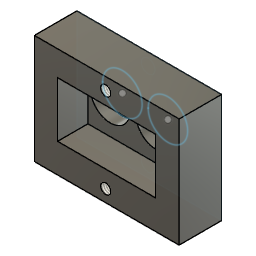
LP8-TAPA v5 (Autodesk Fusion 360 design; units mm, degrees)
Autodesk Fusion 360 part; units mm, degrees
sketch "Boceto1" plane through (0, 0, 0) normal (0, 0, 1) x (1, 0, 0)
  line L0 (0, 0) -> (47.682, 0)
  line L1 (47.682, 0) -> (47.682, 36)
  line L2 (47.682, 36) -> (0, 36)
  line L3 (0, 36) -> (0, 0)
  line L4 (4.2944, 26.5117) -> (42.5805, 26.5117)
  line L5 (42.5805, 26.5117) -> (42.5805, 9.2899)
  line L6 (42.5805, 9.2899) -> (4.2944, 9.2899)
  line L7 (4.2944, 9.2899) -> (4.2944, 26.5117)
  circle A0 centre (23.5, 32) radius 2.25
  circle A1 centre (23.5, 4) radius 2.25
  dimension "d8" = 4.5
  dimension "d10" = 4.5
  constraint horizontal L0
  constraint vertical L1
  constraint horizontal L2
  constraint vertical L3
  constraint coincident L0.start L3.end
  constraint horizontal L4
  constraint vertical L5
  constraint horizontal L6
  constraint vertical L7
  measures "d8" diameter of A0
  measures "d10" diameter of A1
extrude "Extruir1" add sketch "Boceto1" against normal blind 14 contours L0 L1 L2 L3 | L4 L5 L6 L7
sketch "Boceto2" plane through (0, 0, 0) normal (0, 0, 1) x (1, 0, 0)
  circle A0 centre (23.5, 4) radius 2.25
  circle A1 centre (23.5, 32) radius 2.25
  line L0 (0, 36) -> (0, 0)
  line L1 (0, 0) -> (47.682, 0)
  line L2 (47.682, 0) -> (47.682, 36)
  line L3 (47.682, 36) -> (0, 36)
  line L4 (7.6346, 27.7605) -> (39.9467, 27.7605)
  line L5 (39.9467, 27.7605) -> (39.9467, 9.5968)
  line L6 (39.9467, 9.5968) -> (7.6346, 9.5968)
  line L7 (7.6346, 9.5968) -> (7.6346, 27.7605)
  constraint horizontal L4
  constraint vertical L5
  constraint horizontal L6
  constraint vertical L7
extrude "Extruir2" cut sketch "Boceto2" against normal blind 10 contours L4 L5 L6 L7
sketch "Boceto3" plane through (0, 0, -14) normal (0, 0, -1) x (-1, 0, 0)
  circle A0 centre (-23.5, 4) radius 2.25
  circle A1 centre (-23.5, 32) radius 2.25
  line L0 (0, 0) -> (0, 36)
  line L1 (0, 36) -> (-47.682, 36)
  line L2 (-47.682, 36) -> (-47.682, 0)
  line L3 (-47.682, 0) -> (0, 0)
  circle A2 centre (-30, 20) radius 6.5
  circle A3 centre (-15, 20) radius 6.5
  dimension "d25" = 13
  dimension "d26" = 13
  measures "d25" diameter of A2
  measures "d26" diameter of A3
extrude "Extruir3" cut sketch "Boceto3" against normal blind 25 contours A2 | A3
thread "Rosca1" "ISO Metric profile 4.0 M4x0.7 M4x0.7 6H" major diameter 4.1095 minor diameter 3.332 pitch 0.7 angle 60 resizes the face on face at (25.7388, 31.776, -9.3333)
thread "Rosca2" "ISO Metric profile 4.0 M4x0.7 M4x0.7 6H" major diameter 4.1095 minor diameter 3.332 pitch 0.7 angle 60 resizes the face on face at (25.7388, 3.776, -9.3333)
